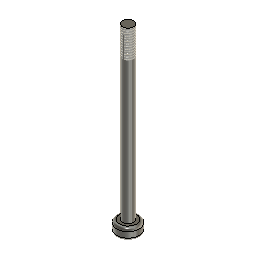
Bolt-M2 (Autodesk Fusion 360 design; units mm, degrees)
part number: 2026-04-30-20-05-40-228
Autodesk Fusion 360 part; units mm, degrees
sketch "Sketch1" plane through (0, 0, 0) normal (0, 0, 1) x (1, 0, 0)
  circle A0 centre (0, 0) radius 2
  dimension "d1" = 4
  constraint coincident A0.centre origin
  measures "d1" diameter of A0
extrude "Extrude1" add sketch "Sketch1" along normal blind 2
sketch "Sketch2" plane through (0, 0, 2) normal (0, 0, 1) x (-1, 0, 0)
  circle A0 centre (0, 0) radius 2
  circle A1 centre (0, 0) radius 1
  dimension "d4" = 2
  constraint coincident A0.centre A1.centre
  measures "d4" diameter of A1
extrude "Extrude2" add sketch "Sketch2" along normal blind 30 contours A1
fillet "Fillet1" radius 0.5 2 edges at (-1.8647, -0.7232, 0) (-1.8647, -0.7232, 2)
thread "Thread3" "ISO Metric profile 2.0 M2x0.4 M2x0.4 6g" major diameter 1.9335 minor diameter 1.478 pitch 0.4 angle 60 resizes the face on face at (-0.995, 0.0996, 22) from (0, 0, 27) to (0, 0, 32)
sketch "Sketch3" plane through (0, 0, 0) normal (0, 0, -1) x (1, 0, 0)
  circle A0 centre (0, 0) radius 1.5
  line L0 (-0.5, 1.25) -> (0.5, 1.25)
  line L1 (0.5, 1.25) -> (0.5, -1.25)
  line L2 (0.5, -1.25) -> (-0.5, -1.25)
  line L3 (-0.5, -1.25) -> (-0.5, 1.25)
  line L4 (-0.5, 1.25) -> (0.5, -1.25) construction
  line L5 (0.5, 1.25) -> (-0.5, -1.25) construction
  line L6 (-1.25, 0.5) -> (1.25, 0.5)
  line L7 (1.25, 0.5) -> (1.25, -0.5)
  line L8 (1.25, -0.5) -> (-1.25, -0.5)
  line L9 (-1.25, -0.5) -> (-1.25, 0.5)
  line L10 (-1.25, 0.5) -> (1.25, -0.5) construction
  line L11 (1.25, 0.5) -> (-1.25, -0.5) construction
  dimension "d17" = 1
  dimension "d18" = 2.5
  dimension "d19" = 2.5
  dimension "d20" = 1
  constraint horizontal L0
  constraint perpendicular L0 L1
  constraint parallel L0 L2
  constraint parallel L1 L3
  constraint coincident L4 A0.centre
  constraint coincident L5 A0.centre
  constraint coincident A0.centre origin
  constraint horizontal L6
  constraint perpendicular L6 L7
  constraint parallel L6 L8
  constraint parallel L7 L9
  constraint coincident L10 A0.centre
  constraint coincident L11 A0.centre
  measures "d17" distance of L1.end L2.end
  measures "d18" distance of L0.end L1.end
  measures "d19" distance of L7.end L8.end
  measures "d20" distance of L6.end L7.end
extrude "Extrude4" cut sketch "Sketch3" against normal blind 1 contours L0 L1 L3 L6 | L1 L3 L6 L8 | L3 L6 L8 L9 | L1 L6 L7 L8 | L1 L2 L3 L8
chamfer "Chamfer1" distance 0.2 angle 45 12 edges at (0, 1.25, 0) (-0.5, 0.875, 0) (0.5, 0.875, 0) (0.875, 0.5, 0) (1.25, 0, 0) (0.875, -0.5, 0) (0.5, -0.875, 0) (0, -1.25, 0) (-0.5, -0.875, 0) (-0.875, 0.5, 0) (-1.25, 0, 0) (-0.875, -0.5, 0)
